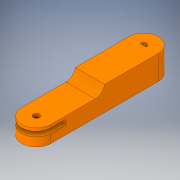
# Autodesk Inventor part: ArmThicker
Saved by Autodesk Inventor 2017 (Build 210142000, 142)
## iProperties
Created: 2017-03-25
Part Number: ArmThicker
Material: Generic
Document SubType Name: Modeling
Designer: Parshant Bombhi
Density: 1 g/cm^3
Appearance: Default
LengthOfArm_Thicker: 7.000 in
Thickness_Thicker: 1.250 in
Author: Parshant Bombhi
Autodesk Inventor part; units mm, degrees
ref_plane "YZ Plane" through (0, 0, 0) normal (1, 0, 0) x (0, 1, 0)
ref_plane "XZ Plane" through (0, 0, 0) normal (0, 1, 0) x (-1, 0, 0)
ref_plane "XY Plane" through (0, 0, 0) normal (0, 0, 1) x (1, 0, 0)
sketch "Sketch1" plane through (0, 0, 0) normal (0, 1, 0) x (-1, 0, 0)
  line L0 (0, -19.05) -> (0, -158.75)
  line L1 (19.05, -177.8) -> (19.05, -177.8)
  line L2 (38.1, -158.75) -> (38.1, -19.05)
  line L3 (19.05, 0) -> (19.05, 0)
  arc A0 (0, -158.75) -> (19.05, -177.8) centre (19.05, -158.75) ccw
  arc A1 (19.05, -177.8) -> (38.1, -158.75) centre (19.05, -158.75) ccw
  arc A2 (38.1, -19.05) -> (19.05, 0) centre (19.05, -19.05) ccw
  arc A3 (19.05, 0) -> (0, -19.05) centre (19.05, -19.05) ccw
  circle A4 centre (19.05, -19.05) radius 3.9688
  circle A5 centre (19.05, -158.75) radius 3.9688
  point P0 (0, 0)
  point P1 (0, -177.8)
  point P2 (38.1, -177.8)
  dimension "d0" = 38.1
  dimension "LengthOfArm_Thicker" = 177.8
  dimension "d2" = 19.05
  dimension "d3" = 7.9375
  dimension "Motor_Shaft_Diameter" = 7.9375
  constraints: 8 end point, 8 point on circle, 8 tangent, 6 centre point, 6 point on line, 3 equal radius, 3 perpendicular, 2 coincident, 1 vertical
  measures "d0" distance of point (0, -177.8) point (38.1, -177.8)
  measures "LengthOfArm_Thicker" distance of point (0, 0) point (0, -177.8)
  measures "d2" radius of A0
  measures "d3" diameter of A4
  measures "Motor_Shaft_Diameter" diameter of A5
extrude "Extrusion1" add sketch "Sketch1" along normal blind 31.75
sketch "Sketch3" plane through (0, 0, -19.05) normal (1, 0, 0) x (0, 0, -1)
  line L0 (-57.15, 11.43) -> (19.05, 11.43)
  line L1 (19.05, 11.43) -> (19.05, 17.78)
  line L2 (19.05, 17.78) -> (-57.15, 17.78)
  line L3 (-57.15, 17.78) -> (-57.15, 11.43)
  line L4 (-19.05, 0) -> (-19.05, 31.75) projected
  line L5 (-57.15, 11.43) -> (19.05, 17.78) construction
  line L6 (19.05, 11.43) -> (-57.15, 17.78) construction
  line L7 (0, 0) -> (-19.05, 0) projected
  line L8 (-19.05, 0) -> (-19.05, 31.75) projected
  line L9 (-19.05, 21.59) -> (69.85, 21.59)
  line L10 (69.85, 21.59) -> (69.85, 31.75)
  line L11 (139.7, 31.75) -> (0, 31.75) projected
  line L12 (0, 31.75) -> (-19.05, 31.75) projected
  line L13 (69.85, 31.75) -> (-19.05, 31.75)
  line L14 (-19.05, 0) -> (-19.05, 31.75) projected
  line L15 (-19.05, 31.75) -> (-19.05, 21.59)
  point P0 (-19.05, 14.605)
  point P1 (-19.05, 14.605)
  dimension "d15" = 6.35
  dimension "d19" = 11.43
  dimension "d20" = 10.16
  dimension "d21" = 88.9
  constraints: 20 end point, 4 perpendicular, 3 midpoint, 2 parallel, 2 point on line, 1 collinear, 1 horizontal
  measures "d15" distance of L0.end L1.end
  measures "d19" distance between parallel lines of L7 L0
  measures "d20" distance between parallel lines of L12 L9
  measures "d21" distance between parallel lines of L10 L4
extrude "Extrusion3" cut sketch "Sketch3" against normal up to next
fillet "Fillet3" radius 12.7 1 edges at (-19.05, 21.59, -88.9)
sketch "Sketch4" plane through (0, 31.75, 0) normal (0, 1, 0) x (1, 0, 0)
  circle A0 centre (-19.05, 158.75) radius 3.9687 projected
  line L0 (-9.6345, 157.9562) -> (-28.4655, 157.9562)
  line L1 (-28.4655, 157.9562) -> (-28.4655, 151.6062)
  line L2 (-28.4655, 151.6062) -> (-9.6345, 151.6062)
  line L3 (-9.6345, 151.6062) -> (-9.6345, 157.9562)
  line L4 (-9.6345, 157.9562) -> (-28.4655, 151.6062) construction
  line L5 (-28.4655, 157.9562) -> (-9.6345, 151.6062) construction
  point P0 (0, 0)
  point P1 (-19.05, 154.7812)
  dimension "d23" = 6.35
  constraints: 12 end point, 2 midpoint, 2 parallel, 1 horizontal, 1 perpendicular, 1 vertical alignment, 1 other
  measures "d23" distance of L0.end L1.end
extrude "Extrusion4" add sketch "Sketch4" against normal up to surface (31.75 mm away) contours L0 A0 | A0 L0 L3 L2 L1 picked at (-18.2787, 156.5235)
equation "\"Thickness_Thicker\" = 2 * Thickness_Thiner"
equation "\"Thickness_Thiner\" = 15.875"
body "Solid1"
